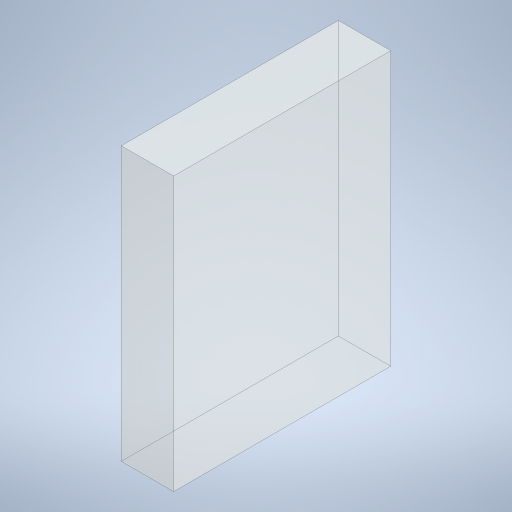
# Autodesk Inventor part: Tankless_Water_Heater
Saved by Autodesk Inventor 2024 (Build 280153020, 153B)
## iProperties
Created: 2023-07-15
Part Number: Tankless_Water_Heater
Material: ABS Plastic
Document SubType Name: Modeling
Designer: Tom
Density: 1.06 g/cm^3
Appearance: Clear
Author: Tom
Autodesk Inventor part; units mm, degrees
ref_plane "YZ Plane" through (0, 0, 0) normal (1, 0, 0) x (0, 1, 0)
ref_plane "XZ Plane" through (0, 0, 0) normal (0, 1, 0) x (-1, 0, 0)
ref_plane "XY Plane" through (0, 0, 0) normal (0, 0, 1) x (1, 0, 0)
sketch "Sketch1" plane through (0, 0, 0) normal (1, 0, 0) x (0, 1, 0)
  line L0 (0, 0) -> (463.55, 0)
  line L1 (463.55, 0) -> (463.55, -368.3)
  line L2 (463.55, -368.3) -> (0, -368.3)
  line L3 (0, -368.3) -> (0, 0)
  dimension "d1" = 463.55
  dimension "d2" = 368.3
  constraints: 8 end point, 2 parallel, 1 horizontal, 1 perpendicular
  measures "d1" distance of L1.end L2.end
  measures "d2" distance of L0.end L1.end
extrude "Extrusion1" add sketch "Sketch1" along normal blind 88.9
body "Solid1"
